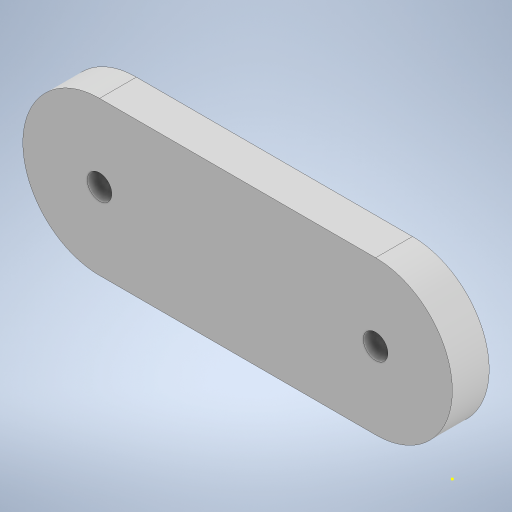
# Autodesk Inventor part: Small Rod
Saved by Autodesk Inventor 2024 (Build 280153000, 153)
## iProperties
Created: 2024-03-08
Part Number: Small Rod
Material: Generic
Document SubType Name: Modeling
Designer: ddcos
Density: 1 g/cm^3
Appearance: Default
Author: ddcos
Autodesk Inventor part; units mm, degrees
ref_plane "YZ Plane" through (0, 0, 0) normal (1, 0, 0) x (0, 1, 0)
ref_plane "XZ Plane" through (0, 0, 0) normal (0, 1, 0) x (-1, 0, 0)
ref_plane "XY Plane" through (0, 0, 0) normal (0, 0, 1) x (1, 0, 0)
sketch "Sketch1" plane through (0, 0, 0) normal (0, 0, 1) x (1, 0, 0)
  line L0 (0, 0) -> (-70, 0)
  line L1 (-70, 0) -> (-70, 25)
  line L2 (-70, 25) -> (0, 25)
  line L3 (0, 25) -> (0, 0)
  dimension "d0" = 25
  dimension "d1" = 70
  constraints: 8 end point, 2 parallel, 1 horizontal, 1 perpendicular
  measures "d0" distance of L2.end L0.start
  measures "d1" distance of L1.end L2.end
extrude "Extrusion1" add sketch "Sketch1" along normal blind 25
sketch "Sketch3" plane through (0, 0, 25) normal (0, 0, 1) x (1, 0, 0)
  line L0 (0, 0) -> (0, 25) projected
  line L1 (-70, 0) -> (0, 0) projected
  circle A0 centre (-12.5, 12.5) radius 12.5 projected
  circle A1 centre (-57.5, 12.5) radius 12.5 projected
  line L2 (-70, 25) -> (-70, 0) projected
  circle A2 centre (-57.5, 12.5) radius 2 projected
  circle A3 centre (-12.5, 12.5) radius 2 projected
  line L3 (0, 25) -> (-70, 25) projected
  point P0 (-12.5, 25)
  point P1 (0, 12.5)
  point P2 (-12.5, 0)
  point P3 (-57.5, 25)
  point P4 (-70, 12.5)
  point P5 (-57.5, 0)
extrude "Extrusion2" cut sketch "Sketch3" against normal blind 25 contours L1 A0 L0 | A0 L3 L0 | L1 L2 A1 | A1 L2 L3 | A2 | A3
sketch "Sketch4" plane through (-57.5, 25, 0) normal (0, 1, 0) x (1, 0, 0)
  line L0 (-12.5, 0) -> (-12.5, -25) projected
  line L1 (57.5, 0) -> (-12.5, 0)
  line L2 (-12.5, 0) -> (-12.5, -19)
  line L3 (-12.5, -19) -> (57.5, -19)
  line L4 (57.5, -19) -> (57.5, 0)
  dimension "d14" = 19
  constraints: 8 end point, 2 parallel, 1 horizontal, 1 perpendicular, 1 point on line
  measures "d14" distance between parallel lines of L1 L3
extrude "Extrusion3" cut sketch "Sketch4" against normal blind 100
sketch "Sketch5" plane through (0, 0, 25) normal (0, 0, 1) x (1, 0, 0)
  point P0 (0, 0)
body "Solid1"
